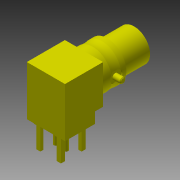
# Autodesk Inventor part: CJT-T-P-HH-RA-TH1
Saved by Autodesk Inventor 2014 SP2 (Build 180246200, 246)
## iProperties
Created: 2018-08-02
Part Number: CJT-T-P-HH-RA-TH1
Material: Generic
Catalog Web Link: www.cadenas.de
Description: CJT-TH Series-Circular RF Twinax Jack, Through-hole
Vendor: SAMTEC
Document SubType Name: Modeling
Designer: psadmin
Manufacturer: SAMTEC
Mass: 0.196031 g
Surface Area: 3.11794 cm^2
Volume: 0.196031 cm^3
Density: 1 g/cm^3
Appearance: PSOLRGB-255-255-0
Category: PARTsolutions
Company: SAMTEC
Title: CJT-T-P-HH-RA-TH1
Author: Cadenas PARTsolutions
Comments: Circular RF Twinax Jack, Through-hole
PSOL_IDENT_0: {$CADENAS_DATA\23d-libs\samtec\modelling\cjt\cjt-th.prj},190 {VTYP=3D},{NB=CJT-T-P-HH-RA-TH1},{LINA=
PSOL_IDENT_1: CJT-T-P-HH-RA-TH1},{NN=CJT-TH Series},{DATE=26.10.2016 12:02:31},{GEOMDATE=19.09.2016 12:10:38},{VER
PSOL_IDENT_2: SION=},{LINEID=10},{WBVAR=PLOPT,ORI},{WBNUMERIC=}  {NB=CJT-T-P-HH-RA-TH1},{LINA=CJT-T-P-HH-RA-TH1},{
PSOL_IDENT_3: KT=DUMMY},{PN=CJT-T-P-HH-RA-TH1},{SERIES=CJT-TH},{GEN=-T: Terminal},{TYPE=-P: PCB},{PLOPT=HH},{PLOPT
PSOL_IDENT_4: ALG= 'HH','-HH: Heavy Gold / Heavy Gold 30 µ\" Au / 50 µ\" Ni Min on Pin 30 µ\" Au / 50 µ\" Ni Min o
PSOL_IDENT_5: n Outer Contact','GF','Non-standard option - Please contact SAMTEC: -GF: Gold / Flash Gold 10 µ\" Au
PSOL_IDENT_6: / 50 µ\" Ni Min on Pin 3 µ\" Au / 50 µ\" Ni Min on Outer Contact' },{ORI=RA},{TERM=-TH1: Through Ho
PSOL_IDENT_7: le}
NN: CJT-TH Series
NT: Circular RF Twinax Jack, Through-hole
NB: CJT-T-P-HH-RA-TH1
NBSYN: $PN.
LINA: CJT-T-P-HH-RA-TH1
PN: CJT-T-P-HH-RA-TH1
SERIES: CJT-TH
GEN: -T: Terminal
TYPE: -P: PCB
PLOPT: -HH: Heavy Gold / Heavy Gold 30 µ" Au / 50 µ" Ni Min on Pin 30 µ" Au / 50 µ" Ni Min on Outer Contact
ORI: -RA: Right Angle
TERM: -TH1: Through Hole
SUPPLIER: SAMTEC
ARTICLENO: CJT-T-P-HH-RA-TH1
BOMINFO: CJT-T-P-HH-RA-TH1
CREATOR: CADENAS GmbH
Autodesk Inventor part; units mm, degrees
sketch "Sketch0" plane through (2.35, 0, 0) normal (1, 0, 0) x (0, 0, -1)
  line L0 (-2.417, -3.8772) -> (6.633, -3.8772)
  line L1 (6.633, -3.8772) -> (6.633, -0.1772)
  line L2 (6.633, -0.1772) -> (2.351, -0.1772)
  line L3 (2.351, -0.1772) -> (2.351, 0.8128)
  line L4 (2.351, 0.8128) -> (-2.417, 0.8128)
  line L5 (-2.417, 0.8128) -> (-2.417, -3.8772)
  constraints: 12 end point
extrude "Extrusion1" add sketch "Sketch0" against normal blind 4.7
sketch "Sketch2" plane through (0, 0, -3.683) normal (0, 0, -1) x (-1, 0, 0)
  line L0 (-2.35, -3.8772) -> (2.35, -3.8772)
  line L1 (2.35, -3.8772) -> (2.35, -0.1772)
  line L2 (2.35, -0.1772) -> (-2.35, -0.1772)
  line L3 (-2.35, -0.1772) -> (-2.35, -3.8772)
  line L4 (0.89, -0.3772) -> (0.89, -0.7888)
  arc A0 (1.2384, -1.1372) -> (0.89, -0.7888) centre (0, -2.0272) ccw
  line L5 (1.2384, -1.1372) -> (1.65, -1.1372)
  line L6 (1.65, -1.1372) -> (1.65, -0.3772)
  line L7 (1.65, -0.3772) -> (0.89, -0.3772)
  line L8 (0.89, -3.6772) -> (1.65, -3.6772)
  line L9 (1.65, -3.6772) -> (1.65, -2.9172)
  line L10 (1.65, -2.9172) -> (1.2384, -2.9172)
  arc A1 (0.89, -3.2656) -> (1.2384, -2.9172) centre (0, -2.0272) ccw
  line L11 (0.89, -3.2656) -> (0.89, -3.6772)
  line L12 (-1.65, -1.1372) -> (-1.2384, -1.1372)
  arc A2 (-0.89, -0.7888) -> (-1.2384, -1.1372) centre (0, -2.0272) ccw
  line L13 (-0.89, -0.7888) -> (-0.89, -0.3772)
  line L14 (-0.89, -0.3772) -> (-1.65, -0.3772)
  line L15 (-1.65, -0.3772) -> (-1.65, -1.1372)
  line L16 (-1.65, -3.6772) -> (-0.89, -3.6772)
  line L17 (-0.89, -3.6772) -> (-0.89, -3.2656)
  arc A3 (-1.2384, -2.9172) -> (-0.89, -3.2656) centre (0, -2.0272) ccw
  line L18 (-1.2384, -2.9172) -> (-1.65, -2.9172)
  line L19 (-1.65, -2.9172) -> (-1.65, -3.6772)
  constraints: 40 end point, 8 point on circle, 4 centre point
sketch "Sketch1" plane through (0, 0, -3.933) normal (0, 0, -1) x (-1, 0, 0)
  line L0 (-3.3075, -4.3481) -> (3.6398, -4.3481)
  line L1 (3.6398, -4.3481) -> (3.6398, 0.0953)
  line L2 (3.6398, 0.0953) -> (-3.3075, 0.0953)
  line L3 (-3.3075, 0.0953) -> (-3.3075, -4.3481)
  line L4 (1.015, -0.5022) -> (1.015, -0.889)
  arc A0 (1.1382, -1.0122) -> (1.015, -0.889) centre (0, -2.0272) ccw
  line L5 (1.1382, -1.0122) -> (1.525, -1.0122)
  line L6 (1.525, -1.0122) -> (1.525, -0.5022)
  line L7 (1.525, -0.5022) -> (1.015, -0.5022)
  line L8 (1.015, -3.5522) -> (1.525, -3.5522)
  line L9 (1.525, -3.5522) -> (1.525, -3.0422)
  line L10 (1.525, -3.0422) -> (1.1382, -3.0422)
  arc A1 (1.015, -3.1654) -> (1.1382, -3.0422) centre (0, -2.0272) ccw
  line L11 (1.015, -3.1654) -> (1.015, -3.5522)
  line L12 (-1.525, -0.5022) -> (-1.525, -1.0122)
  line L13 (-1.525, -1.0122) -> (-1.1382, -1.0122)
  arc A2 (-1.015, -0.889) -> (-1.1382, -1.0122) centre (0, -2.0272) ccw
  line L14 (-1.015, -0.889) -> (-1.015, -0.5022)
  line L15 (-1.015, -0.5022) -> (-1.525, -0.5022)
  line L16 (-1.525, -3.5522) -> (-1.015, -3.5522)
  line L17 (-1.015, -3.5522) -> (-1.015, -3.1654)
  arc A3 (-1.1382, -3.0422) -> (-1.015, -3.1654) centre (0, -2.0272) ccw
  line L18 (-1.1382, -3.0422) -> (-1.525, -3.0422)
  line L19 (-1.525, -3.0422) -> (-1.525, -3.5522)
  constraints: 40 end point, 8 point on circle, 4 centre point
extrude "Extrusion2" cut sketch "Sketch1" along normal blind 2.7
sketch "Sketch3" plane through (0, 0, -3.683) normal (0, 0, -1) x (-1, 0, 0)
  circle A0 centre (0.635, -2.0272) radius 0.255
  constraints: 1 centre point
extrude "Extrusion3" cut sketch "Sketch2" along normal blind 2.95
sketch "Sketch4" plane through (0, 0, -3.683) normal (0, 0, -1) x (-1, 0, 0)
  circle A0 centre (-0.635, -2.0272) radius 0.255
  constraints: 1 centre point
extrude "Extrusion4" add sketch "Sketch3" along normal blind 2.7104
sketch "Sketch5" plane through (0, 0, 0) normal (1, 0, 0) x (0, 0, -1)
  line L0 (0, 3.6828) -> (0, 0.8128)
  line L1 (0, 0.8128) -> (-2.35, 0.8128)
  line L2 (-2.35, 0.8128) -> (-2.35, 1.8878)
  arc A0 (-2.35, 1.8878) -> (-2.35, 3.0378) centre (-4.6766, 2.4628) ccw
  line L3 (-2.35, 3.0378) -> (-2.35, 3.6828)
  line L4 (-2.35, 3.6828) -> (-1.97, 3.6828)
  line L5 (-1.97, 3.6828) -> (-1.97, 6.9828)
  line L6 (-1.97, 6.9828) -> (-1.65, 6.9828)
  line L7 (-1.65, 6.9828) -> (-1.575, 6.5575)
  line L8 (-1.575, 6.5575) -> (-1.575, 3.6828)
  line L9 (-1.575, 3.6828) -> (0, 3.6828)
  line L10 (0, 3.6828) -> (0, 0.8128)
  constraints: 22 end point, 2 point on circle, 1 centre point
extrude "Extrusion5" add sketch "Sketch4" along normal blind 2.7104
sketch "Sketch6" plane through (0, 0, 0) normal (0, 0, 1) x (1, 0, 0)
  line L0 (-1.2208, 7.9291) -> (-0.4483, 6.5911)
  arc A0 (-0.38, 6.3361) -> (-0.4483, 6.5911) centre (-0.89, 6.3361) ccw
  line L1 (-0.38, 6.3361) -> (-0.38, 4.2628)
  arc A1 (-0.38, 4.2628) -> (0.38, 4.2628) centre (0, 4.2628) ccw
  line L2 (0.38, 4.2628) -> (0.38, 6.3361)
  arc A2 (0.4483, 6.5911) -> (0.38, 6.3361) centre (0.89, 6.3361) ccw
  line L3 (0.4483, 6.5911) -> (1.2208, 7.9291)
  line L4 (1.2208, 7.9291) -> (-1.2208, 7.9291)
  constraints: 10 end point, 6 point on circle, 3 centre point
revolve "Revolution1" add sketch "Sketch5" angle 360 about axis through (0, 3.6828, 0) along (0, 1, 0)
sketch "Sketch7" plane through (2.2, 0, 0) normal (1, 0, 0) x (0, 0, -1)
  circle A0 centre (0, 2.4628) radius 0.75
  constraints: 1 centre point
extrude "Extrusion6" cut sketch "Sketch6" against normal blind 3
sketch "Sketch8" plane through (-2.2, 0, 0) normal (-1, 0, 0) x (0, 0, 1)
  circle A0 centre (0, 2.4628) radius 0.75
  constraints: 1 centre point
extrude "Extrusion7" cut sketch "Sketch7" along normal blind 0.15
sketch "Sketch9" plane through (0, 0, 0) normal (0, 0, 1) x (1, 0, 0)
  line L0 (3.175, 2.4628) -> (-3.175, 2.4628)
  line L1 (-3.175, 2.4628) -> (-3.175, 2.7128)
  line L2 (-3.175, 2.7128) -> (-3.075, 2.8128)
  line L3 (-3.075, 2.8128) -> (3.075, 2.8128)
  line L4 (3.075, 2.8128) -> (3.175, 2.7128)
  line L5 (3.175, 2.7128) -> (3.175, 2.4628)
  line L6 (3.175, 2.4628) -> (-3.175, 2.4628)
  constraints: 14 end point
extrude "Extrusion8" cut sketch "Sketch8" along normal blind 0.15
sketch "Sketch10" plane through (0, 0, 0) normal (0, 0, 1) x (1, 0, 0)
  line L0 (0.635, 6.2728) -> (0.635, 3.6828)
  line L1 (0.635, 3.6828) -> (0.445, 3.6828)
  line L2 (0.445, 3.6828) -> (0.445, 6.0828)
  arc A0 (0.635, 6.2728) -> (0.445, 6.0828) centre (0.635, 6.0828) ccw
  line L3 (0.635, 6.2728) -> (0.635, 3.6828)
  constraints: 8 end point, 2 point on circle, 1 centre point
revolve "Revolution2" add sketch "Sketch9" angle 360 about axis through (3.175, 2.4628, 0) along (1, 0, 0)
sketch "Sketch11" plane through (0, 0, 0) normal (0, 0, 1) x (1, 0, 0)
  line L0 (-0.635, 6.2728) -> (-0.635, 3.6828)
  line L1 (-0.635, 3.6828) -> (-0.825, 3.6828)
  line L2 (-0.825, 3.6828) -> (-0.825, 6.0828)
  arc A0 (-0.635, 6.2728) -> (-0.825, 6.0828) centre (-0.635, 6.0828) ccw
  line L3 (-0.635, 6.2728) -> (-0.635, 3.6828)
  constraints: 8 end point, 2 point on circle, 1 centre point
revolve "Revolution3" add sketch "Sketch10" angle 360 about axis through (0.635, 6.2728, 0) along (0, 1, 0)
revolve "Revolution4" add sketch "Sketch11" angle 360 about axis through (-0.635, 6.2728, 0) along (0, 1, 0)
ref_plane "fh1_XY" through (0, 6.9828, 0) normal (0, 0, 1) x (1, 0, 0)
ref_plane "fh1_YZ" through (0, 6.9828, 0) normal (1, 0, 0) x (0, 1, 0)
ref_plane "fh1_ZX" through (0, 6.9828, 0) normal (0, 1, 0) x (0, 0, 1)
body "Solid1"
